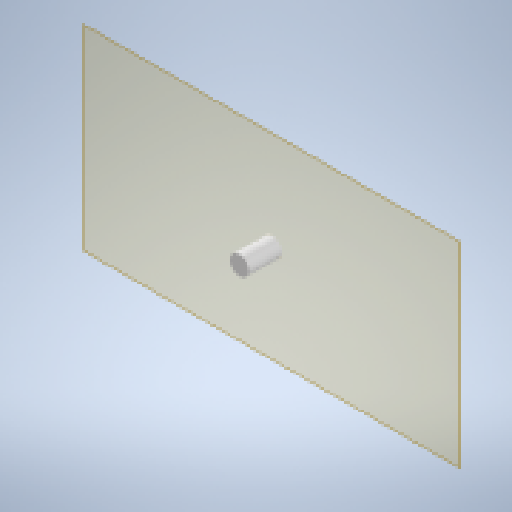
# Autodesk Inventor part: GEAR_SHAFT1
Saved by Autodesk Inventor 2024 (Build 280153000, 153)
## iProperties
Created: 2024-04-16
Part Number: GEAR_SHAFT1
Material: Generic
Document SubType Name: Modeling
Designer: teeta
Density: 1 g/cm^3
Appearance: Default
Author: teeta
Autodesk Inventor part; units mm, degrees
ref_plane "YZ Plane" through (0, 0, 0) normal (1, 0, 0) x (0, 1, 0)
ref_plane "XZ Plane" through (0, 0, 0) normal (0, 1, 0) x (-1, 0, 0)
ref_plane "XY Plane" through (0, 0, 0) normal (0, 0, 1) x (1, 0, 0)
ref_plane "Work Plane1" through (0, 0, 0) normal (0, 0, 1) x (1, 0, 0)
sketch "Sketch1" plane through (0, 0, 0) normal (0, 0, 1) x (1, 0, 0)
  line L0 (-187.5, 97.5) -> (187.5, 97.5) projected
  line L1 (-187.5, -97.5) -> (-187.5, 97.5) projected
  line L2 (187.5, -97.5) -> (-187.5, -97.5) projected
  line L3 (187.5, 97.5) -> (187.5, -97.5) projected
  line L4 (0, -97.5) -> (0, 97.5) construction
  line L5 (-187.5, 0) -> (187.5, 0) construction
  circle A0 centre (0, 16.075) radius 10.2232
  line L6 (-404.725, 6.075) -> (404.725, 6.075)
  line L7 (-404.725, 26.075) -> (404.725, 26.075)
  line L8 (0, 26.075) -> (0, 6.075)
  dimension "d0" = 20.4464
  constraints: 10 end point, 7 midpoint, 2 horizontal, 1 centre point, 1 coincident, 4 other
  measures "d0" diameter of A0
extrude "Extrusion1" add sketch "Sketch1" along normal blind 35.75 contours L7 L8 L6 A0 | A0 L7 | A0 L6 L8 L7 | L6 A0
body "Solid1"
